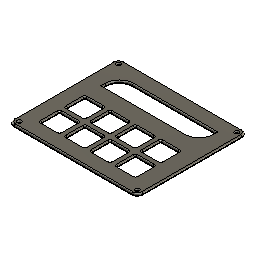
Final (Autodesk Fusion 360 archive; units mm, degrees)
design "Case_Lid"
Autodesk Fusion 360 part; units mm, degrees
(part 1 of 2)
sketch "plate-2025-12-06T19_36_10.325Z" plane through (0, 0, 0) normal (0, 0, 1) x (1, 0, 0)
  line L0 (3.275, -2.525) -> (15.775, -2.525)
  line L1 (3.275, -16.525) -> (15.775, -16.525)
  line L2 (2.525, -3.275) -> (2.525, -15.775)
  line L3 (16.525, -3.275) -> (16.525, -15.775)
  arc A0 (3.275, -2.525) -> (2.525, -3.275) centre (3.275, -3.275) ccw
  arc A1 (16.525, -3.275) -> (15.775, -2.525) centre (15.775, -3.275) ccw
  arc A2 (2.525, -15.775) -> (3.275, -16.525) centre (3.275, -15.775) ccw
  arc A3 (15.775, -16.525) -> (16.525, -15.775) centre (15.775, -15.775) ccw
  line L4 (22.325, -2.525) -> (34.825, -2.525)
  line L5 (22.325, -16.525) -> (34.825, -16.525)
  line L6 (21.575, -3.275) -> (21.575, -15.775)
  line L7 (35.575, -3.275) -> (35.575, -15.775)
  arc A4 (22.325, -2.525) -> (21.575, -3.275) centre (22.325, -3.275) ccw
  arc A5 (35.575, -3.275) -> (34.825, -2.525) centre (34.825, -3.275) ccw
  arc A6 (21.575, -15.775) -> (22.325, -16.525) centre (22.325, -15.775) ccw
  arc A7 (34.825, -16.525) -> (35.575, -15.775) centre (34.825, -15.775) ccw
  line L8 (41.375, -2.525) -> (53.875, -2.525)
  line L9 (41.375, -16.525) -> (53.875, -16.525)
  line L10 (40.625, -3.275) -> (40.625, -15.775)
  line L11 (54.625, -3.275) -> (54.625, -15.775)
  arc A8 (41.375, -2.525) -> (40.625, -3.275) centre (41.375, -3.275) ccw
  arc A9 (54.625, -3.275) -> (53.875, -2.525) centre (53.875, -3.275) ccw
  arc A10 (40.625, -15.775) -> (41.375, -16.525) centre (41.375, -15.775) ccw
  arc A11 (53.875, -16.525) -> (54.625, -15.775) centre (53.875, -15.775) ccw
  line L12 (60.425, -2.525) -> (72.925, -2.525)
  line L13 (60.425, -16.525) -> (72.925, -16.525)
  line L14 (59.675, -3.275) -> (59.675, -15.775)
  line L15 (73.675, -3.275) -> (73.675, -15.775)
  arc A12 (60.425, -2.525) -> (59.675, -3.275) centre (60.425, -3.275) ccw
  arc A13 (73.675, -3.275) -> (72.925, -2.525) centre (72.925, -3.275) ccw
  arc A14 (59.675, -15.775) -> (60.425, -16.525) centre (60.425, -15.775) ccw
  arc A15 (72.925, -16.525) -> (73.675, -15.775) centre (72.925, -15.775) ccw
  line L16 (3.275, -21.575) -> (15.775, -21.575)
  line L17 (3.275, -35.575) -> (15.775, -35.575)
  line L18 (2.525, -22.325) -> (2.525, -34.825)
  line L19 (16.525, -22.325) -> (16.525, -34.825)
  arc A16 (3.275, -21.575) -> (2.525, -22.325) centre (3.275, -22.325) ccw
  arc A17 (16.525, -22.325) -> (15.775, -21.575) centre (15.775, -22.325) ccw
  arc A18 (2.525, -34.825) -> (3.275, -35.575) centre (3.275, -34.825) ccw
  arc A19 (15.775, -35.575) -> (16.525, -34.825) centre (15.775, -34.825) ccw
  line L20 (22.325, -21.575) -> (34.825, -21.575)
  line L21 (22.325, -35.575) -> (34.825, -35.575)
  line L22 (21.575, -22.325) -> (21.575, -34.825)
  line L23 (35.575, -22.325) -> (35.575, -34.825)
  arc A20 (22.325, -21.575) -> (21.575, -22.325) centre (22.325, -22.325) ccw
  arc A21 (35.575, -22.325) -> (34.825, -21.575) centre (34.825, -22.325) ccw
  arc A22 (21.575, -34.825) -> (22.325, -35.575) centre (22.325, -34.825) ccw
  arc A23 (34.825, -35.575) -> (35.575, -34.825) centre (34.825, -34.825) ccw
  line L24 (41.375, -21.575) -> (53.875, -21.575)
  line L25 (41.375, -35.575) -> (53.875, -35.575)
  line L26 (40.625, -22.325) -> (40.625, -34.825)
  line L27 (54.625, -22.325) -> (54.625, -34.825)
  arc A24 (41.375, -21.575) -> (40.625, -22.325) centre (41.375, -22.325) ccw
  arc A25 (54.625, -22.325) -> (53.875, -21.575) centre (53.875, -22.325) ccw
  arc A26 (40.625, -34.825) -> (41.375, -35.575) centre (41.375, -34.825) ccw
  arc A27 (53.875, -35.575) -> (54.625, -34.825) centre (53.875, -34.825) ccw
  line L28 (60.425, -21.575) -> (72.925, -21.575)
  line L29 (60.425, -35.575) -> (72.925, -35.575)
  line L30 (59.675, -22.325) -> (59.675, -34.825)
  line L31 (73.675, -22.325) -> (73.675, -34.825)
  arc A28 (60.425, -21.575) -> (59.675, -22.325) centre (60.425, -22.325) ccw
  arc A29 (73.675, -22.325) -> (72.925, -21.575) centre (72.925, -22.325) ccw
  arc A30 (59.675, -34.825) -> (60.425, -35.575) centre (60.425, -34.825) ccw
  arc A31 (72.925, -35.575) -> (73.675, -34.825) centre (72.925, -34.825) ccw
  line L32 (-9.861, 35.425) -> (87.139, 35.425)
  line L33 (87.139, 35.425) -> (87.139, -47.575)
  line L34 (87.139, -47.575) -> (-9.861, -47.575)
  line L35 (-9.861, -47.575) -> (-9.861, 35.425)
  line L36 (12.525, 23.425) -> (74.753, 23.425)
  line L37 (74.753, 23.425) -> (74.753, 21.425)
  line L38 (64.753, 11.425) -> (2.525, 11.425)
  line L39 (2.525, 11.425) -> (2.525, 13.425)
  arc A32 (12.525, 23.425) -> (2.525, 13.425) centre (12.525, 13.425) ccw
  arc A33 (64.753, 11.425) -> (74.753, 21.425) centre (64.753, 21.425) ccw
  circle A34 centre (-5.861, 31.425) radius 1.6
  circle A35 centre (83.139, 31.425) radius 1.6
  circle A36 centre (83.139, -43.575) radius 1.6
  circle A37 centre (-5.861, -43.575) radius 1.6
  point P0 (74.753, 11.425)
  dimension "d1" = 97
  dimension "d2" = 83
  dimension "d3" = 12.386
  dimension "d4" = 12
  dimension "d5" = 0
  dimension "d6" = 12.386
  dimension "d7" = 12.386
  dimension "d8" = 12
  dimension "d9" = 12
  dimension "d10" = 10
  dimension "d11" = 10
  dimension "d12" = 3.2
  dimension "d13" = 4
  dimension "d14" = 4
  dimension "d15" = 3.2
  dimension "d16" = 4
  dimension "d17" = 4
  dimension "d18" = 3.2
  dimension "d19" = 3.2
  dimension "d20" = 4
  dimension "d21" = 4
  dimension "d22" = 4
  dimension "d23" = 4
  constraint horizontal L32
  constraint vertical L33
  constraint horizontal L34
  constraint vertical L35
  constraint horizontal L36
  constraint vertical L37
  constraint horizontal L38
  constraint vertical L39
  constraint tangent L36 A32
  constraint tangent L39 A32
  constraint coincident P0 L38
  constraint tangent L37 A33
  constraint tangent L38 A33
  measures "d1" distance of L32.start L32.end
  measures "d2" distance of L32.start L34.end
  measures "d3" distance of L18 L35
  measures "d4" distance of L17 L34
  measures "d5" distance of L2 L39
  measures "d6" distance of L33 L37
  measures "d7" distance of L35 L39
  measures "d8" distance of L36.end P0
  measures "d9" distance of L32 L36
  measures "d10" radius of A32
  measures "d11" radius of A33
  measures "d12" diameter of A34
  measures "d13" distance of L32 A34.centre
  measures "d14" distance of L35 A34.centre
  measures "d15" diameter of A35
  measures "d16" distance of L33 A35.centre
  measures "d17" distance of L32 A35.centre
  measures "d18" diameter of A37
  measures "d19" diameter of A36
  measures "d20" distance of L34 A36.centre
  measures "d21" distance of L33 A36.centre
  measures "d22" distance of L34 A37.centre
  measures "d23" distance of L35 A37.centre
extrude "Extrude1" add sketch "plate-2025-12-06T19_36_10.325Z" along normal blind 1.5
fillet "Fillet2" radius 4.3 4 edges at (-9.861, 35.425, 0.75) (87.139, 35.425, 0.75) (-9.861, -47.575, 0.75) (87.139, -47.575, 0.75)
fillet "Fillet1" radius 1 74 edges at (21.7947, -35.3553, 1.5) (21.575, -28.575, 1.5) (21.7947, -21.7947, 1.5) (28.575, -21.575, 1.5) (35.3553, -21.7947, 1.5) (35.575, -28.575, 1.5) (35.3553, -35.3553, 1.5) (28.575, -35.575, 1.5) (2.525, -28.575, 1.5) (2.7447, -21.7947, 1.5) (9.525, -21.575, 1.5) (16.3053, -21.7947, 1.5) (16.525, -28.575, 1.5) (16.3053, -35.3553, 1.5) (9.525, -35.575, 1.5) (2.7447, -35.3553, 1.5) (28.575, -2.525, 1.5) (35.3553, -2.7447, 1.5) (35.575, -9.525, 1.5) (35.3553, -16.3053, 1.5) (28.575, -16.525, 1.5) (21.7947, -16.3053, 1.5) (21.575, -9.525, 1.5) (21.7947, -2.7447, 1.5) (74.753, 22.425, 1.5) (71.8241, 14.3539, 1.5) (33.639, 11.425, 1.5) (2.525, 12.425, 1.5) (5.4539, 20.4961, 1.5) (43.639, 23.425, 1.5) (87.139, -6.075, 1.5) (38.639, 35.425, 1.5) (-9.861, -6.075, 1.5) (38.639, -47.575, 1.5) (16.3053, -2.7447, 1.5) (16.525, -9.525, 1.5) (16.3053, -16.3053, 1.5) (9.525, -16.525, 1.5) (2.7447, -16.3053, 1.5) (2.525, -9.525, 1.5) (2.7447, -2.7447, 1.5) (9.525, -2.525, 1.5) (40.8447, -35.3553, 1.5) (40.625, -28.575, 1.5) (40.8447, -21.7947, 1.5) (47.625, -21.575, 1.5) (54.4053, -21.7947, 1.5) (54.625, -28.575, 1.5) (54.4053, -35.3553, 1.5) (47.625, -35.575, 1.5) (47.625, -2.525, 1.5) (54.4053, -2.7447, 1.5) (54.625, -9.525, 1.5) (54.4053, -16.3053, 1.5) (47.625, -16.525, 1.5) (40.8447, -16.3053, 1.5) (40.625, -9.525, 1.5) (40.8447, -2.7447, 1.5) (59.675, -9.525, 1.5) (59.8947, -2.7447, 1.5) (66.675, -2.525, 1.5) (73.4553, -2.7447, 1.5) (73.675, -9.525, 1.5) (73.4553, -16.3053, 1.5) (66.675, -16.525, 1.5) (59.8947, -16.3053, 1.5) (59.8947, -35.3553, 1.5) (59.675, -28.575, 1.5) (59.8947, -21.7947, 1.5) (66.675, -21.575, 1.5) (73.4553, -21.7947, 1.5) (73.675, -28.575, 1.5) (73.4553, -35.3553, 1.5) (66.675, -35.575, 1.5)
equation "d1 = 8 mm + 8 mm + 81 mm"
equation "d2 = 8 mm + 8 mm + 67 mm"
equation "d3 = 8 mm + 4.386 mm"
equation "d4 = 8 mm + 4 mm"

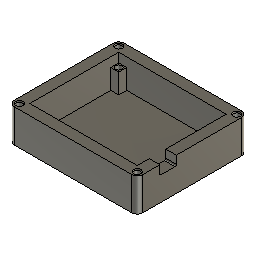
design "Case_Base"
Autodesk Fusion 360 part; units mm, degrees
sketch "Sketch1" plane through (0, 0, 0) normal (0, 0, 1) x (1, 0, 0) in component "Hackpad Case"
  line L0 (1, 47.0118) -> (82, 47.0118)
  line L1 (82, 47.0118) -> (82, -19.9882)
  line L2 (82, -19.9882) -> (1, -19.9882)
  line L3 (1, -19.9882) -> (1, 47.0118)
  line L4 (-7, 55.0118) -> (90, 55.0118)
  line L5 (90, 55.0118) -> (90, -27.9882)
  line L6 (90, -27.9882) -> (-7, -27.9882)
  line L7 (-7, -27.9882) -> (-7, 55.0118)
  circle A0 centre (-3, 51.0118) radius 2.35
  circle A1 centre (86, 51.0118) radius 2.35
  circle A2 centre (-3, -23.9882) radius 2.35
  circle A3 centre (86, -23.9882) radius 2.35
  circle A4 centre (4, 44.0118) radius 2.35
  line L8 (1, 47.0118) -> (7, 47.0118)
  line L9 (7, 47.0118) -> (7, 41.0118)
  line L10 (7, 41.0118) -> (1, 41.0118)
  line L11 (1, 41.0118) -> (1, 47.0118)
  circle A5 centre (79, 44.0118) radius 2.35
  line L12 (82, 47.0118) -> (76, 47.0118)
  line L13 (76, 47.0118) -> (76, 41.0118)
  line L14 (76, 41.0118) -> (82, 41.0118)
  line L15 (82, 41.0118) -> (82, 47.0118)
  circle A6 centre (4, -16.9882) radius 2.35
  line L16 (1, -19.9882) -> (7, -19.9882)
  line L17 (7, -19.9882) -> (7, -13.9882)
  line L18 (7, -13.9882) -> (1, -13.9882)
  line L19 (1, -13.9882) -> (1, -19.9882)
  line L20 (82, -19.9882) -> (76, -19.9882)
  line L21 (76, -19.9882) -> (76, -13.9882)
  line L22 (76, -13.9882) -> (82, -13.9882)
  line L23 (82, -13.9882) -> (82, -19.9882)
  circle A7 centre (79, -16.9882) radius 2.35
  point P0 (-24.0837, 40.5707)
  dimension "d1" = 81
  dimension "d2" = 67
  dimension "d3" = 8
  dimension "d4" = 8
  dimension "d5" = 8
  dimension "d6" = 8
  dimension "d7" = 4.7
  dimension "d8" = 4
  dimension "d9" = 4
  dimension "d10" = 4.7
  dimension "d11" = 4
  dimension "d12" = 4
  dimension "d13" = 4.7
  dimension "d14" = 4
  dimension "d15" = 4
  dimension "d16" = 4.7
  dimension "d17" = 4
  dimension "d18" = 4
  dimension "d22" = 4.7
  dimension "d23" = 3
  dimension "d24" = 3
  dimension "d25" = 6
  dimension "d26" = 6
  dimension "d27" = 4.7
  dimension "d28" = 6
  dimension "d29" = 6
  dimension "d30" = 3
  dimension "d31" = 3
  dimension "d32" = 4.7
  dimension "d33" = 6
  dimension "d34" = 6
  dimension "d35" = 3
  dimension "d36" = 3
  dimension "d37" = 6
  dimension "d38" = 6
  dimension "d39" = 4.7
  dimension "d40" = 3
  dimension "d41" = 3
  constraint horizontal L0
  constraint vertical L1
  constraint horizontal L2
  constraint vertical L3
  constraint horizontal L4
  constraint vertical L5
  constraint horizontal L6
  constraint vertical L7
  constraint horizontal L8
  constraint vertical L9
  constraint horizontal L10
  constraint vertical L11
  constraint horizontal L12
  constraint vertical L13
  constraint horizontal L14
  constraint vertical L15
  constraint horizontal L16
  constraint vertical L17
  constraint horizontal L18
  constraint vertical L19
  constraint horizontal L20
  constraint vertical L21
  constraint horizontal L22
  constraint vertical L23
  measures "d1" distance of L0.start L0.end
  measures "d2" distance of L0.start L2.end
  measures "d3" distance of L0 L4
  measures "d4" distance of L2 L6
  measures "d5" distance of L1 L5
  measures "d6" distance of L3 L7
  measures "d7" diameter of A0
  measures "d8" distance of L7 A0.centre
  measures "d9" distance of L4 A0.centre
  measures "d10" diameter of A1
  measures "d11" distance of L4 A1.centre
  measures "d12" distance of L5 A1.centre
  measures "d13" diameter of A2
  measures "d14" distance of L7 A2.centre
  measures "d15" distance of L6 A2.centre
  measures "d16" diameter of A3
  measures "d17" distance of L5 A3.centre
  measures "d18" distance of L6 A3.centre
  measures "d22" diameter of A4
  measures "d23" distance of L3 A4.centre
  measures "d24" distance of L0 A4.centre
  measures "d25" distance of L8.end L9.end
  measures "d26" distance of L9.end L10.end
  measures "d27" diameter of A5
  measures "d28" distance of L13.end L14.end
  measures "d29" distance of L12.end L13.end
  measures "d30" distance of A5.centre L12
  measures "d31" distance of L1 A5.centre
  measures "d32" diameter of A6
  measures "d33" distance of L17.end L18.end
  measures "d34" distance of L16.end L17.end
  measures "d35" distance of L2 A6.centre
  measures "d36" distance of A6.centre L19
  measures "d37" distance of L21.end L22.end
  measures "d38" distance of L20.end L21.end
  measures "d39" diameter of A7
  measures "d40" distance of L23 A7.centre
  measures "d41" distance of L2 A7.centre
extrude "Extrude1" add sketch "Sketch1" along normal blind 3.1 contours L0 L3 L8 L9 L10 L11 | L0 L1 L2 L3 L9 L10 L13 L14 L17 L18 L21 L22 | L0 L1 L12 L13 L14 L15 | L2 L3 L16 L17 L18 L19 | L1 L2 L20 L21 L22 L23 | L4 L5 L6 L7 | A0 | A1 | A2 | A3 | A4 | A5 | A6 | A7 in component "Hackpad Case"
extrude "Extrude2" add sketch "Sketch1" along normal blind 25 contours L4 L5 L6 L7 in component "Hackpad Case"
extrude "Extrude3" add sketch "Sketch1" along normal blind 18 contours L0 L3 L8 L9 L10 L11 | L0 L1 L12 L13 L14 L15 | L2 L3 L16 L17 L18 L19 | L1 L2 L20 L21 L22 L23 in component "Hackpad Case"
fillet "Fillet1" radius 4.3 4 edges at (90, -27.9882, 12.5) (90, 55.0118, 12.5) (-7, -27.9882, 12.5) (-7, 55.0118, 12.5) in component "Hackpad Case"
sketch "Sketch2" plane through (0, 0, 25) normal (0, 0, 1) x (-1, 0, 0) in component "Hackpad Case"
  circle A0 centre (3, 23.9882) radius 2.35
  circle A1 centre (3, -51.0118) radius 2.35
  line L0 (-82, -47.0118) -> (-82, 19.9882)
  line L1 (-82, 19.9882) -> (-1, 19.9882)
  line L2 (-1, 19.9882) -> (-1, -47.0118)
  line L3 (-1, -47.0118) -> (-82, -47.0118)
  circle A2 centre (-86, -51.0118) radius 2.35
  circle A3 centre (-86, 23.9882) radius 2.35
  arc A4 (2.7, -55.0118) -> (7, -50.7118) centre (2.7, -50.7118) ccw
  line L4 (7, -50.7118) -> (7, 23.6882)
  arc A5 (7, 23.6882) -> (2.7, 27.9882) centre (2.7, 23.6882) ccw
  line L5 (2.7, 27.9882) -> (-85.7, 27.9882)
  arc A6 (-85.7, 27.9882) -> (-90, 23.6882) centre (-85.7, 23.6882) ccw
  line L6 (-90, 23.6882) -> (-90, -50.7118)
  arc A7 (-90, -50.7118) -> (-85.7, -55.0118) centre (-85.7, -50.7118) ccw
  line L7 (-85.7, -55.0118) -> (2.7, -55.0118)
  line L8 (-82, -1.5118) -> (-90, -1.5118)
  line L9 (-90, -1.5118) -> (-90, 10.9882)
  line L10 (-90, 10.9882) -> (-82, 10.9882)
  line L11 (-82, 10.9882) -> (-82, -1.5118)
  dimension "d54" = 9
  dimension "d55" = 12.5
  constraint horizontal L8
  constraint vertical L9
  constraint horizontal L10
  constraint vertical L11
  constraint coincident L6 L9.end
  constraint coincident L0 L8.start
  measures "d54" distance of L1 L10
  measures "d55" distance of L8.end L9.end
extrude "Extrude4" cut sketch "Sketch2" against normal up to surface (7 mm away) contours L0 L6 L8 L9 L10 L11 in component "Hackpad Case"
fillet "Fillet2" radius 1 2 edges at (86, -10.9882, 18) (86, 1.5118, 18) in component "Hackpad Case"
chamfer "Chamfer1" distance 0.4 distance2 0.8 4 edges at (-5.191, -23.1384, 25) (-5.191, 51.8616, 25) (83.809, 51.8616, 25) (83.809, -23.1384, 25) measured on face at (84.6667, 16.6784, 25) measured on face at (84.6667, 16.6784, 25) measured on face at (84.6667, 16.6784, 25) measured on face at (84.6667, 16.6784, 25) in component "Hackpad Case"
sketch "Sketch1 (2)" plane through (0, 0, 0) normal (0, 0, -1) x (1, 0, 0)
  arc A0 (-7, -50.7118) -> (-2.7, -55.0118) centre (-2.7, -50.7118) ccw
  line L0 (-2.7, -55.0118) -> (85.7, -55.0118)
  arc A1 (85.7, -55.0118) -> (90, -50.7118) centre (85.7, -50.7118) ccw
  line L1 (90, -50.7118) -> (90, 23.6882)
  arc A2 (90, 23.6882) -> (85.7, 27.9882) centre (85.7, 23.6882) ccw
  line L2 (85.7, 27.9882) -> (-2.7, 27.9882)
  arc A3 (-2.7, 27.9882) -> (-7, 23.6882) centre (-2.7, 23.6882) ccw
  line L3 (-7, 23.6882) -> (-7, -50.7118)
  line L4 (86.6421, -50.8903) -> (39.0171, -50.8903)
  line L5 (39.0171, -50.8903) -> (39.0171, -35.0153)
  line L6 (39.0171, -35.0153) -> (86.6421, -35.0153)
  line L7 (86.6421, -35.0153) -> (86.6421, -50.8903)
  line L8 (54.9424, -39.6039) -> (57.298, -40.1975)
  line L9 (57.298, -40.1975) -> (57.2281, -40.4746)
  line L10 (57.2281, -40.4746) -> (54.7859, -39.859)
  spline S0 degree 3 poles (54.7859, -39.859) (54.5214, -40.2569) (54.1891, -40.6039) (53.7828, -40.8953) knots 0 0 0 0 1 1 1 1
  line L11 (53.7828, -40.8953) -> (53.1572, -43.2146)
  line L12 (53.1572, -43.2146) -> (51.4906, -41.7411)
  spline S1 degree 3 poles (51.4906, -41.7411) (49.6525, -42.1963) (47.9026, -42.1789) (46.2353, -41.7201) knots 0 0 0 0 1 1 1 1
  line L13 (46.2353, -41.7201) -> (44.5832, -43.0742)
  line L14 (44.5832, -43.0742) -> (44.2797, -41.1871)
  spline S2 degree 3 poles (44.2797, -41.1871) (43.932, -40.8137) (43.6708, -40.4314) (43.4786, -40.0419) knots 0 0 0 0 1 1 1 1
  line L15 (43.4786, -40.0419) -> (42.3068, -40.4518)
  line L16 (42.3068, -40.4518) -> (42.2124, -40.1822)
  line L17 (42.2124, -40.1822) -> (43.3603, -39.7805)
  spline S3 degree 3 poles (43.3603, -39.7805) (43.2125, -39.4227) (43.1191, -39.0592) (43.067, -38.6915) knots 0 0 0 0 1 1 1 1
  line L18 (43.067, -38.6915) -> (40.8577, -38.6743)
  line L19 (40.8577, -38.6743) -> (40.8598, -38.3886)
  line L20 (40.8598, -38.3886) -> (43.0346, -38.4054)
  spline S4 degree 3 poles (43.0346, -38.4054) (43.0153, -38.1788) (43.0102, -37.9506) (43.0164, -37.7212) knots 0 0 0 0 1 1 1 1
  line L21 (43.0164, -37.7212) -> (43.0203, -37.5772)
  line L22 (43.0203, -37.5772) -> (43.3083, -37.585)
  line L23 (43.3083, -37.585) -> (43.3044, -37.729)
  spline S5 degree 3 poles (43.3044, -37.729) (43.2982, -37.9566) (43.3038, -38.1829) (43.3244, -38.4077) knots 0 0 0 0 1 1 1 1
  line L24 (43.3244, -38.4077) -> (45.1702, -38.4221)
  line L25 (45.1702, -38.4221) -> (45.168, -38.7078)
  line L26 (45.168, -38.7078) -> (43.3591, -38.6938)
  spline S6 degree 3 poles (43.3591, -38.6938) (43.41, -39.0283) (43.498, -39.359) (43.6339, -39.6848) knots 0 0 0 0 1 1 1 1
  line L27 (43.6339, -39.6848) -> (45.2416, -39.1224)
  line L28 (45.2416, -39.1224) -> (45.336, -39.3921)
  line L29 (45.336, -39.3921) -> (43.7538, -39.9456)
  spline S7 degree 3 poles (43.7538, -39.9456) (43.9379, -40.3117) (44.1878, -40.671) (44.5195, -41.0217) knots 0 0 0 0 1 1 1 1
  line L30 (44.5195, -41.0217) -> (44.55, -41.0539)
  line L31 (44.55, -41.0539) -> (44.788, -42.5338)
  line L32 (44.788, -42.5338) -> (46.1689, -41.4022)
  line L33 (46.1689, -41.4022) -> (46.2413, -41.4227)
  spline S8 degree 3 poles (46.2413, -41.4227) (47.9053, -41.894) (49.6541, -41.911) (51.4936, -41.4433) knots 0 0 0 0 1 1 1 1
  line L34 (51.4936, -41.4433) -> (51.5675, -41.4245)
  line L35 (51.5675, -41.4245) -> (53, -42.6911)
  line L36 (53, -42.6911) -> (53.5317, -40.7195)
  line L37 (53.5317, -40.7195) -> (53.5747, -40.6895)
  spline S9 degree 3 poles (53.5747, -40.6895) (53.9407, -40.434) (54.2431, -40.1306) (54.4875, -39.7839) knots 0 0 0 0 1 1 1 1
  line L38 (54.4875, -39.7839) -> (53.0484, -39.4212)
  line L39 (53.0484, -39.4212) -> (53.1182, -39.144)
  line L40 (53.1182, -39.144) -> (54.6514, -39.5305)
  spline S10 degree 3 poles (54.6514, -39.5305) (54.8036, -39.2737) (54.9279, -38.9961) (55.0266, -38.6993) knots 0 0 0 0 1 1 1 1
  line L41 (55.0266, -38.6993) -> (53.8649, -38.9048)
  line L42 (53.8649, -38.9048) -> (53.8152, -38.6233)
  line L43 (53.8152, -38.6233) -> (55.1177, -38.393)
  spline S11 degree 3 poles (55.1177, -38.393) (55.1323, -38.3375) (55.1461, -38.2814) (55.1591, -38.2248) knots 0 0 0 0 1 1 1 1
  line L44 (55.1591, -38.2248) -> (55.1915, -38.0844)
  line L45 (55.1915, -38.0844) -> (55.4722, -38.1489)
  line L46 (55.4722, -38.1489) -> (55.44, -38.2894)
  spline S12 degree 3 poles (55.44, -38.2894) (55.4362, -38.3056) (55.4323, -38.3218) (55.4285, -38.338) knots 0 0 0 0 1 1 1 1
  line L47 (55.4285, -38.338) -> (56.726, -38.1084)
  line L48 (56.726, -38.1084) -> (56.7757, -38.3898)
  line L49 (56.7757, -38.3898) -> (55.3467, -38.6427)
  spline S13 degree 3 poles (55.3467, -38.6427) (55.2437, -38.9867) (55.1096, -39.3077) (54.9424, -39.6039) knots 0 0 0 0 1 1 1 1
  spline S14 degree 3 poles (82.8096, -44.1615) (83.112, -44.1615) (83.3711, -44.2087) (83.5869, -44.303) knots 0 0 0 0 1 1 1 1
  spline S15 degree 3 poles (83.5869, -44.303) (83.8028, -44.3974) (83.9627, -44.5346) (84.0667, -44.7146) knots 0 0 0 0 1 1 1 1
  spline S16 degree 3 poles (84.0667, -44.7146) (84.1707, -44.8947) (84.207, -45.1131) (84.1755, -45.3701) knots 0 0 0 0 1 1 1 1
  line L50 (84.1755, -45.3701) -> (83.486, -45.3701)
  spline S17 degree 3 poles (83.486, -45.3701) (83.5035, -45.1656) (83.4431, -45.0127) (83.3051, -44.9113) knots 0 0 0 0 1 1 1 1
  spline S18 degree 3 poles (83.3051, -44.9113) (83.167, -44.81) (82.9878, -44.7593) (82.7676, -44.7593) knots 0 0 0 0 1 1 1 1
  spline S19 degree 3 poles (82.7676, -44.7593) (82.5369, -44.7593) (82.3399, -44.8108) (82.1764, -44.9139) knots 0 0 0 0 1 1 1 1
  spline S20 degree 3 poles (82.1764, -44.9139) (82.013, -45.017) (81.9173, -45.1534) (81.8894, -45.3229) knots 0 0 0 0 1 1 1 1
  spline S21 degree 3 poles (81.8894, -45.3229) (81.8632, -45.475) (81.9082, -45.5895) (82.0244, -45.6664) knots 0 0 0 0 1 1 1 1
  spline S22 degree 3 poles (82.0244, -45.6664) (82.1406, -45.7432) (82.301, -45.8096) (82.5055, -45.8656) knots 0 0 0 0 1 1 1 1
  line L51 (82.5055, -45.8656) -> (82.9302, -45.9809)
  spline S23 degree 3 poles (82.9302, -45.9809) (83.229, -46.0596) (83.4594, -46.1823) (83.621, -46.3493) knots 0 0 0 0 1 1 1 1
  spline S24 degree 3 poles (83.621, -46.3493) (83.7827, -46.5162) (83.8408, -46.7422) (83.7954, -47.027) knots 0 0 0 0 1 1 1 1
  spline S25 degree 3 poles (83.7954, -47.027) (83.7586, -47.2577) (83.6682, -47.4596) (83.524, -47.6326) knots 0 0 0 0 1 1 1 1
  spline S26 degree 3 poles (83.524, -47.6326) (83.3798, -47.8057) (83.1958, -47.9403) (82.9722, -48.0364) knots 0 0 0 0 1 1 1 1
  spline S27 degree 3 poles (82.9722, -48.0364) (82.7484, -48.1325) (82.4993, -48.1806) (82.225, -48.1806) knots 0 0 0 0 1 1 1 1
  spline S28 degree 3 poles (82.225, -48.1806) (81.9505, -48.1806) (81.7124, -48.1325) (81.5105, -48.0364) knots 0 0 0 0 1 1 1 1
  spline S29 degree 3 poles (81.5105, -48.0364) (81.3086, -47.9403) (81.1579, -47.8079) (81.0582, -47.6391) knots 0 0 0 0 1 1 1 1
  spline S30 degree 3 poles (81.0582, -47.6391) (80.9587, -47.4706) (80.9245, -47.2769) (80.956, -47.0585) knots 0 0 0 0 1 1 1 1
  line L52 (80.956, -47.0585) -> (81.6324, -47.0585)
  spline S31 degree 3 poles (81.6324, -47.0585) (81.6219, -47.2245) (81.6753, -47.3538) (81.7923, -47.4465) knots 0 0 0 0 1 1 1 1
  spline S32 degree 3 poles (81.7923, -47.4465) (81.9095, -47.5392) (82.0738, -47.5855) (82.2852, -47.5855) knots 0 0 0 0 1 1 1 1
  spline S33 degree 3 poles (82.2852, -47.5855) (82.5072, -47.5855) (82.6885, -47.5369) (82.8292, -47.4399) knots 0 0 0 0 1 1 1 1
  spline S34 degree 3 poles (82.8292, -47.4399) (82.9699, -47.343) (83.0534, -47.221) (83.0796, -47.0742) knots 0 0 0 0 1 1 1 1
  spline S35 degree 3 poles (83.0796, -47.0742) (83.0989, -46.9658) (83.0809, -46.8767) (83.0258, -46.8068) knots 0 0 0 0 1 1 1 1
  spline S36 degree 3 poles (83.0258, -46.8068) (82.9708, -46.7369) (82.8957, -46.6805) (82.8004, -46.6377) knots 0 0 0 0 1 1 1 1
  spline S37 degree 3 poles (82.8004, -46.6377) (82.7052, -46.5948) (82.606, -46.5603) (82.5029, -46.5341) knots 0 0 0 0 1 1 1 1
  line L53 (82.5029, -46.5341) -> (82.1542, -46.4398)
  spline S38 degree 3 poles (82.1542, -46.4398) (81.9707, -46.3943) (81.7984, -46.3274) (81.6377, -46.2392) knots 0 0 0 0 1 1 1 1
  spline S39 degree 3 poles (81.6377, -46.2392) (81.4769, -46.1509) (81.3528, -46.0325) (81.2654, -45.8839) knots 0 0 0 0 1 1 1 1
  spline S40 degree 3 poles (81.2654, -45.8839) (81.1779, -45.7354) (81.1535, -45.5466) (81.192, -45.3177) knots 0 0 0 0 1 1 1 1
  spline S41 degree 3 poles (81.192, -45.3177) (81.2479, -44.9733) (81.4148, -44.6945) (81.6928, -44.4814) knots 0 0 0 0 1 1 1 1
  spline S42 degree 3 poles (81.6928, -44.4814) (81.9707, -44.2681) (82.3429, -44.1615) (82.8096, -44.1615) knots 0 0 0 0 1 1 1 1
  line L54 (79.383, -48.1282) -> (80.0305, -44.2218)
  line L55 (80.0305, -44.2218) -> (80.7306, -44.2218)
  line L56 (80.7306, -44.2218) -> (80.0829, -48.1282)
  line L57 (80.0829, -48.1282) -> (79.383, -48.1282)
  line L58 (79.244, -44.2218) -> (78.5965, -48.1282)
  line L59 (78.5965, -48.1282) -> (77.8964, -48.1282)
  line L60 (77.8964, -48.1282) -> (78.447, -44.8117)
  line L61 (78.447, -44.8117) -> (76.722, -44.8117)
  line L62 (76.722, -44.8117) -> (76.8189, -44.2218)
  line L63 (76.8189, -44.2218) -> (79.244, -44.2218)
  line L64 (76.4702, -44.2218) -> (74.4593, -48.1282)
  line L65 (74.4593, -48.1282) -> (73.5706, -48.1282)
  line L66 (73.5706, -48.1282) -> (72.8234, -44.2218)
  line L67 (72.8234, -44.2218) -> (73.5628, -44.2218)
  line L68 (73.5628, -44.2218) -> (73.7332, -45.1891)
  line L69 (73.7332, -45.1891) -> (75.1961, -45.1891)
  line L70 (75.1961, -45.1891) -> (75.6758, -44.2218)
  line L71 (75.6758, -44.2218) -> (76.4702, -44.2218)
  line L72 (74.9155, -45.7528) -> (73.8327, -45.7528)
  line L73 (73.8327, -45.7528) -> (73.9193, -46.251)
  spline S43 degree 3 poles (73.9193, -46.251) (73.9455, -46.4205) (73.9721, -46.6167) (73.9993, -46.8396) knots 0 0 0 0 1 1 1 1
  spline S44 degree 3 poles (73.9993, -46.8396) (74.0263, -47.0624) (74.0538, -47.3101) (74.0819, -47.5828) knots 0 0 0 0 1 1 1 1
  spline S45 degree 3 poles (74.0819, -47.5828) (74.1937, -47.3171) (74.2981, -47.0733) (74.3951, -46.8514) knots 0 0 0 0 1 1 1 1
  spline S46 degree 3 poles (74.3951, -46.8514) (74.4921, -46.6294) (74.5835, -46.4292) (74.6691, -46.251) knots 0 0 0 0 1 1 1 1
  line L74 (74.6691, -46.251) -> (74.9155, -45.7528)
  spline S47 degree 3 poles (70.9462, -44.1615) (71.2486, -44.1615) (71.5077, -44.2087) (71.7236, -44.303) knots 0 0 0 0 1 1 1 1
  spline S48 degree 3 poles (71.7236, -44.303) (71.9394, -44.3974) (72.0994, -44.5346) (72.2034, -44.7146) knots 0 0 0 0 1 1 1 1
  spline S49 degree 3 poles (72.2034, -44.7146) (72.3073, -44.8947) (72.3436, -45.1131) (72.3121, -45.3701) knots 0 0 0 0 1 1 1 1
  line L75 (72.3121, -45.3701) -> (71.6226, -45.3701)
  spline S50 degree 3 poles (71.6226, -45.3701) (71.6401, -45.1656) (71.5798, -45.0127) (71.4418, -44.9113) knots 0 0 0 0 1 1 1 1
  spline S51 degree 3 poles (71.4418, -44.9113) (71.3037, -44.81) (71.1246, -44.7593) (70.9043, -44.7593) knots 0 0 0 0 1 1 1 1
  spline S52 degree 3 poles (70.9043, -44.7593) (70.6735, -44.7593) (70.4765, -44.8108) (70.313, -44.9139) knots 0 0 0 0 1 1 1 1
  spline S53 degree 3 poles (70.313, -44.9139) (70.1497, -45.017) (70.0539, -45.1534) (70.026, -45.3229) knots 0 0 0 0 1 1 1 1
  spline S54 degree 3 poles (70.026, -45.3229) (69.9998, -45.475) (70.0448, -45.5895) (70.161, -45.6664) knots 0 0 0 0 1 1 1 1
  spline S55 degree 3 poles (70.161, -45.6664) (70.2773, -45.7432) (70.4376, -45.8096) (70.6421, -45.8656) knots 0 0 0 0 1 1 1 1
  line L76 (70.6421, -45.8656) -> (71.0668, -45.9809)
  spline S56 degree 3 poles (71.0668, -45.9809) (71.3658, -46.0596) (71.596, -46.1823) (71.7577, -46.3493) knots 0 0 0 0 1 1 1 1
  spline S57 degree 3 poles (71.7577, -46.3493) (71.9193, -46.5162) (71.9774, -46.7422) (71.932, -47.027) knots 0 0 0 0 1 1 1 1
  spline S58 degree 3 poles (71.932, -47.027) (71.8953, -47.2577) (71.8049, -47.4596) (71.6606, -47.6326) knots 0 0 0 0 1 1 1 1
  spline S59 degree 3 poles (71.6606, -47.6326) (71.5164, -47.8057) (71.3325, -47.9403) (71.1088, -48.0364) knots 0 0 0 0 1 1 1 1
  spline S60 degree 3 poles (71.1088, -48.0364) (70.8851, -48.1325) (70.636, -48.1806) (70.3616, -48.1806) knots 0 0 0 0 1 1 1 1
  spline S61 degree 3 poles (70.3616, -48.1806) (70.0872, -48.1806) (69.849, -48.1325) (69.6471, -48.0364) knots 0 0 0 0 1 1 1 1
  spline S62 degree 3 poles (69.6471, -48.0364) (69.4453, -47.9403) (69.2946, -47.8079) (69.1949, -47.6391) knots 0 0 0 0 1 1 1 1
  spline S63 degree 3 poles (69.1949, -47.6391) (69.0953, -47.4706) (69.0612, -47.2769) (69.0927, -47.0585) knots 0 0 0 0 1 1 1 1
  line L77 (69.0927, -47.0585) -> (69.769, -47.0585)
  spline S64 degree 3 poles (69.769, -47.0585) (69.7586, -47.2245) (69.8119, -47.3538) (69.929, -47.4465) knots 0 0 0 0 1 1 1 1
  spline S65 degree 3 poles (69.929, -47.4465) (70.0461, -47.5392) (70.2104, -47.5855) (70.4219, -47.5855) knots 0 0 0 0 1 1 1 1
  spline S66 degree 3 poles (70.4219, -47.5855) (70.6439, -47.5855) (70.8252, -47.5369) (70.966, -47.4399) knots 0 0 0 0 1 1 1 1
  spline S67 degree 3 poles (70.966, -47.4399) (71.1066, -47.343) (71.1901, -47.221) (71.2163, -47.0742) knots 0 0 0 0 1 1 1 1
  spline S68 degree 3 poles (71.2163, -47.0742) (71.2355, -46.9658) (71.2176, -46.8767) (71.1626, -46.8068) knots 0 0 0 0 1 1 1 1
  spline S69 degree 3 poles (71.1626, -46.8068) (71.1075, -46.7369) (71.0323, -46.6805) (70.9371, -46.6377) knots 0 0 0 0 1 1 1 1
  spline S70 degree 3 poles (70.9371, -46.6377) (70.8418, -46.5948) (70.7426, -46.5603) (70.6395, -46.5341) knots 0 0 0 0 1 1 1 1
  line L78 (70.6395, -46.5341) -> (70.2908, -46.4398)
  spline S71 degree 3 poles (70.2908, -46.4398) (70.1073, -46.3943) (69.9352, -46.3274) (69.7743, -46.2392) knots 0 0 0 0 1 1 1 1
  spline S72 degree 3 poles (69.7743, -46.2392) (69.6135, -46.1509) (69.4894, -46.0325) (69.4021, -45.8839) knots 0 0 0 0 1 1 1 1
  spline S73 degree 3 poles (69.4021, -45.8839) (69.3147, -45.7354) (69.2902, -45.5466) (69.3286, -45.3177) knots 0 0 0 0 1 1 1 1
  spline S74 degree 3 poles (69.3286, -45.3177) (69.3846, -44.9733) (69.5515, -44.6945) (69.8294, -44.4814) knots 0 0 0 0 1 1 1 1
  spline S75 degree 3 poles (69.8294, -44.4814) (70.1073, -44.2681) (70.4796, -44.1615) (70.9462, -44.1615) knots 0 0 0 0 1 1 1 1
  line L79 (68.2642, -46.5472) -> (68.0754, -48.1282)
  line L80 (68.0754, -48.1282) -> (67.4017, -48.1282)
  line L81 (67.4017, -48.1282) -> (67.732, -46.5472)
  line L82 (67.732, -46.5472) -> (68.2642, -46.5472)
  line L83 (84.2201, -37.7252) -> (83.5726, -41.6315)
  line L84 (83.5726, -41.6315) -> (82.8594, -41.6315)
  line L85 (82.8594, -41.6315) -> (83.0534, -40.4727)
  line L86 (83.0534, -40.4727) -> (83.1897, -39.7123)
  spline S76 degree 3 poles (83.1897, -39.7123) (83.0849, -39.8382) (82.9756, -39.961) (82.862, -40.0808) knots 0 0 0 0 1 1 1 1
  spline S77 degree 3 poles (82.862, -40.0808) (82.7484, -40.2005) (82.6225, -40.3277) (82.4845, -40.4622) knots 0 0 0 0 1 1 1 1
  line L87 (82.4845, -40.4622) -> (81.2654, -41.6315)
  line L88 (81.2654, -41.6315) -> (80.3556, -41.6315)
  line L89 (80.3556, -41.6315) -> (82.1358, -39.9404)
  line L90 (82.1358, -39.9404) -> (80.977, -37.7252)
  line L91 (80.977, -37.7252) -> (81.753, -37.7252)
  line L92 (81.753, -37.7252) -> (82.6628, -39.5106)
  line L93 (82.6628, -39.5106) -> (83.313, -38.9102)
  line L94 (83.313, -38.9102) -> (83.5069, -37.7252)
  line L95 (83.5069, -37.7252) -> (84.2201, -37.7252)
  line L96 (80.4448, -37.7252) -> (79.7972, -41.6315)
  line L97 (79.7972, -41.6315) -> (77.2593, -41.6315)
  line L98 (77.2593, -41.6315) -> (77.359, -41.0442)
  line L99 (77.359, -41.0442) -> (79.1968, -41.0442)
  line L100 (79.1968, -41.0442) -> (79.3699, -39.9877)
  line L101 (79.3699, -39.9877) -> (77.6684, -39.9877)
  line L102 (77.6684, -39.9877) -> (77.7653, -39.4082)
  line L103 (77.7653, -39.4082) -> (79.4695, -39.4082)
  line L104 (79.4695, -39.4082) -> (79.6478, -38.3123)
  line L105 (79.6478, -38.3123) -> (77.7995, -38.3123)
  line L106 (77.7995, -38.3123) -> (77.8964, -37.7252)
  line L107 (77.8964, -37.7252) -> (80.4448, -37.7252)
  line L108 (75.9957, -37.7252) -> (75.744, -39.2378)
  line L109 (75.744, -39.2378) -> (76.79, -41.6315)
  line L110 (76.79, -41.6315) -> (76.0114, -41.6315)
  line L111 (76.0114, -41.6315) -> (75.5186, -40.3993)
  spline S78 degree 3 poles (75.5186, -40.3993) (75.48, -40.3032) (75.4456, -40.2101) (75.415, -40.1201) knots 0 0 0 0 1 1 1 1
  spline S79 degree 3 poles (75.415, -40.1201) (75.3844, -40.0301) (75.3569, -39.9309) (75.3324, -39.8225) knots 0 0 0 0 1 1 1 1
  spline S80 degree 3 poles (75.3324, -39.8225) (75.2712, -39.9343) (75.2109, -40.0352) (75.1515, -40.1253) knots 0 0 0 0 1 1 1 1
  spline S81 degree 3 poles (75.1515, -40.1253) (75.092, -40.2153) (75.0283, -40.3066) (74.9601, -40.3993) knots 0 0 0 0 1 1 1 1
  line L112 (74.9601, -40.3993) -> (74.0739, -41.6315)
  line L113 (74.0739, -41.6315) -> (73.2219, -41.6315)
  line L114 (73.2219, -41.6315) -> (75.0466, -39.2378)
  line L115 (75.0466, -39.2378) -> (75.2957, -37.7252)
  line L116 (75.2957, -37.7252) -> (75.9957, -37.7252)
  line L117 (73.3451, -37.7252) -> (72.6976, -41.6315)
  line L118 (72.6976, -41.6315) -> (71.2372, -41.6315)
  spline S82 degree 3 poles (71.2372, -41.6315) (70.9384, -41.6315) (70.6963, -41.576) (70.5111, -41.465) knots 0 0 0 0 1 1 1 1
  spline S83 degree 3 poles (70.5111, -41.465) (70.3257, -41.3541) (70.1964, -41.2011) (70.123, -41.0062) knots 0 0 0 0 1 1 1 1
  spline S84 degree 3 poles (70.123, -41.0062) (70.0496, -40.8113) (70.0338, -40.5898) (70.0758, -40.3416) knots 0 0 0 0 1 1 1 1
  spline S85 degree 3 poles (70.0758, -40.3416) (70.116, -40.0916) (70.2051, -39.8692) (70.3432, -39.6743) knots 0 0 0 0 1 1 1 1
  spline S86 degree 3 poles (70.3432, -39.6743) (70.4813, -39.4795) (70.6627, -39.3261) (70.8872, -39.2143) knots 0 0 0 0 1 1 1 1
  spline S87 degree 3 poles (70.8872, -39.2143) (71.1119, -39.1024) (71.3744, -39.0464) (71.6751, -39.0464) knots 0 0 0 0 1 1 1 1
  line L119 (71.6751, -39.0464) -> (72.4275, -39.0464)
  line L120 (72.4275, -39.0464) -> (72.6451, -37.7252)
  line L121 (72.6451, -37.7252) -> (73.3451, -37.7252)
  line L122 (72.3305, -39.6232) -> (71.6751, -39.6232)
  spline S88 degree 3 poles (71.6751, -39.6232) (71.4042, -39.6232) (71.1975, -39.6914) (71.0551, -39.8278) knots 0 0 0 0 1 1 1 1
  spline S89 degree 3 poles (71.0551, -39.8278) (70.9126, -39.964) (70.8247, -40.1345) (70.7916, -40.3389) knots 0 0 0 0 1 1 1 1
  spline S90 degree 3 poles (70.7916, -40.3389) (70.7565, -40.5452) (70.789, -40.7144) (70.8885, -40.8463) knots 0 0 0 0 1 1 1 1
  spline S91 degree 3 poles (70.8885, -40.8463) (70.9882, -40.9782) (71.1726, -41.0442) (71.4418, -41.0442) knots 0 0 0 0 1 1 1 1
  line L123 (71.4418, -41.0442) -> (72.0972, -41.0442)
  line L124 (72.0972, -41.0442) -> (72.3305, -39.6232)
  line L125 (70.574, -37.7252) -> (68.5631, -41.6315)
  line L126 (68.5631, -41.6315) -> (67.6744, -41.6315)
  line L127 (67.6744, -41.6315) -> (66.9272, -37.7252)
  line L128 (66.9272, -37.7252) -> (67.6664, -37.7252)
  line L129 (67.6664, -37.7252) -> (67.8368, -38.6925)
  line L130 (67.8368, -38.6925) -> (69.2997, -38.6925)
  line L131 (69.2997, -38.6925) -> (69.7795, -37.7252)
  line L132 (69.7795, -37.7252) -> (70.574, -37.7252)
  line L133 (69.0193, -39.2562) -> (67.9365, -39.2562)
  line L134 (67.9365, -39.2562) -> (68.023, -39.7543)
  spline S92 degree 3 poles (68.023, -39.7543) (68.0492, -39.9239) (68.0759, -40.1201) (68.1029, -40.3429) knots 0 0 0 0 1 1 1 1
  spline S93 degree 3 poles (68.1029, -40.3429) (68.1301, -40.5657) (68.1576, -40.8135) (68.1855, -41.0861) knots 0 0 0 0 1 1 1 1
  spline S94 degree 3 poles (68.1855, -41.0861) (68.2974, -40.8205) (68.4019, -40.5767) (68.4989, -40.3547) knots 0 0 0 0 1 1 1 1
  spline S95 degree 3 poles (68.4989, -40.3547) (68.5958, -40.1328) (68.6872, -39.9326) (68.7728, -39.7543) knots 0 0 0 0 1 1 1 1
  line L135 (68.7728, -39.7543) -> (69.0193, -39.2562)
  line L136 (64.9844, -37.7252) -> (66.4054, -37.7252)
  line L137 (66.4054, -37.7252) -> (65.7578, -41.6315)
  line L138 (65.7578, -41.6315) -> (64.4653, -41.6315)
  spline S96 degree 3 poles (64.4653, -41.6315) (64.0773, -41.6315) (63.7522, -41.5533) (63.49, -41.3968) knots 0 0 0 0 1 1 1 1
  spline S97 degree 3 poles (63.49, -41.3968) (63.2278, -41.2404) (63.0417, -41.0162) (62.9316, -40.7243) knots 0 0 0 0 1 1 1 1
  spline S98 degree 3 poles (62.9316, -40.7243) (62.8215, -40.4325) (62.8005, -40.0838) (62.8687, -39.6783) knots 0 0 0 0 1 1 1 1
  spline S99 degree 3 poles (62.8687, -39.6783) (62.9701, -39.0665) (63.1999, -38.5881) (63.5582, -38.2429) knots 0 0 0 0 1 1 1 1
  spline S100 degree 3 poles (63.5582, -38.2429) (63.9165, -37.8977) (64.3919, -37.7252) (64.9844, -37.7252) knots 0 0 0 0 1 1 1 1
  line L139 (65.6058, -38.3307) -> (65.0212, -38.3307)
  spline S101 degree 3 poles (65.0212, -38.3307) (64.1944, -38.3307) (63.7076, -38.7816) (63.5608, -39.6836) knots 0 0 0 0 1 1 1 1
  spline S102 degree 3 poles (63.5608, -39.6836) (63.4123, -40.5784) (63.7408, -41.0259) (64.5466, -41.0259) knots 0 0 0 0 1 1 1 1
  line L140 (64.5466, -41.0259) -> (65.1601, -41.0259)
  line L141 (65.1601, -41.0259) -> (65.6058, -38.3307)
  line L142 (57.4731, -48.1436) -> (57.4731, -45.3714)
  line L143 (57.4731, -45.3714) -> (57.7969, -45.3714)
  line L144 (57.7969, -45.3714) -> (57.7969, -47.7977)
  line L145 (57.7969, -47.7977) -> (57.7987, -47.7977)
  line L146 (57.7987, -47.7977) -> (58.489, -47.3399)
  line L147 (58.489, -47.3399) -> (58.489, -47.6822)
  line L148 (58.489, -47.6822) -> (57.7969, -48.1436)
  line L149 (57.7969, -48.1436) -> (57.4731, -48.1436)
  line L150 (57.0396, -45.3714) -> (57.0396, -45.6523)
  line L151 (57.0396, -45.6523) -> (56.0534, -46.5528)
  spline S103 degree 3 poles (56.0534, -46.5528) (55.9356, -46.6608) (55.8398, -46.7557) (55.766, -46.8375) knots 0 0 0 0 1 1 1 1
  spline S104 degree 3 poles (55.766, -46.8375) (55.6922, -46.9194) (55.638, -46.9995) (55.6032, -47.0775) knots 0 0 0 0 1 1 1 1
  spline S105 degree 3 poles (55.6032, -47.0775) (55.5685, -47.1557) (55.5511, -47.2419) (55.5511, -47.3362) knots 0 0 0 0 1 1 1 1
  spline S106 degree 3 poles (55.5511, -47.3362) (55.5511, -47.5074) (55.6017, -47.6426) (55.7027, -47.7418) knots 0 0 0 0 1 1 1 1
  spline S107 degree 3 poles (55.7027, -47.7418) (55.8038, -47.841) (55.9424, -47.8906) (56.1185, -47.8906) knots 0 0 0 0 1 1 1 1
  spline S108 degree 3 poles (56.1185, -47.8906) (56.3084, -47.8906) (56.4554, -47.8327) (56.5596, -47.7167) knots 0 0 0 0 1 1 1 1
  spline S109 degree 3 poles (56.5596, -47.7167) (56.6637, -47.6007) (56.7158, -47.4441) (56.7158, -47.2469) knots 0 0 0 0 1 1 1 1
  line L152 (56.7158, -47.2469) -> (57.0284, -47.2469)
  spline S110 degree 3 poles (57.0284, -47.2469) (57.0284, -47.4317) (56.9909, -47.5948) (56.9159, -47.7362) knots 0 0 0 0 1 1 1 1
  spline S111 degree 3 poles (56.9159, -47.7362) (56.8408, -47.8777) (56.735, -47.9883) (56.5986, -48.0683) knots 0 0 0 0 1 1 1 1
  spline S112 degree 3 poles (56.5986, -48.0683) (56.4622, -48.1484) (56.3028, -48.1883) (56.1205, -48.1883) knots 0 0 0 0 1 1 1 1
  spline S113 degree 3 poles (56.1205, -48.1883) (55.9468, -48.1883) (55.7936, -48.1527) (55.6608, -48.0814) knots 0 0 0 0 1 1 1 1
  spline S114 degree 3 poles (55.6608, -48.0814) (55.5281, -48.0101) (55.424, -47.9114) (55.3482, -47.7855) knots 0 0 0 0 1 1 1 1
  spline S115 degree 3 poles (55.3482, -47.7855) (55.2726, -47.6596) (55.2347, -47.5142) (55.2347, -47.3492) knots 0 0 0 0 1 1 1 1
  spline S116 degree 3 poles (55.2347, -47.3492) (55.2347, -47.1706) (55.2841, -47.0062) (55.3827, -46.8561) knots 0 0 0 0 1 1 1 1
  spline S117 degree 3 poles (55.3827, -46.8561) (55.4813, -46.7061) (55.6324, -46.5385) (55.8358, -46.3537) knots 0 0 0 0 1 1 1 1
  line L153 (55.8358, -46.3537) -> (56.5856, -45.6728)
  line L154 (56.5856, -45.6728) -> (56.5856, -45.669)
  line L155 (56.5856, -45.669) -> (55.2181, -45.669)
  line L156 (55.2181, -45.669) -> (55.2181, -45.3714)
  line L157 (55.2181, -45.3714) -> (57.0396, -45.3714)
  spline S118 degree 3 poles (54.6412, -45.3398) (54.7058, -45.3398) (54.7606, -45.3623) (54.8059, -45.4077) knots 0 0 0 0 1 1 1 1
  spline S119 degree 3 poles (54.8059, -45.4077) (54.8512, -45.453) (54.8738, -45.5079) (54.8738, -45.5723) knots 0 0 0 0 1 1 1 1
  spline S120 degree 3 poles (54.8738, -45.5723) (54.8738, -45.6381) (54.8512, -45.6933) (54.8059, -45.7379) knots 0 0 0 0 1 1 1 1
  spline S121 degree 3 poles (54.8059, -45.7379) (54.7606, -45.7826) (54.7058, -45.8049) (54.6412, -45.8049) knots 0 0 0 0 1 1 1 1
  spline S122 degree 3 poles (54.6412, -45.8049) (54.5755, -45.8049) (54.5203, -45.7826) (54.4756, -45.7379) knots 0 0 0 0 1 1 1 1
  spline S123 degree 3 poles (54.4756, -45.7379) (54.4311, -45.6933) (54.4087, -45.6381) (54.4087, -45.5723) knots 0 0 0 0 1 1 1 1
  spline S124 degree 3 poles (54.4087, -45.5723) (54.4087, -45.5079) (54.4311, -45.453) (54.4756, -45.4077) knots 0 0 0 0 1 1 1 1
  spline S125 degree 3 poles (54.4756, -45.4077) (54.5203, -45.3623) (54.5755, -45.3398) (54.6412, -45.3398) knots 0 0 0 0 1 1 1 1
  spline S126 degree 3 poles (53.1732, -45.3342) (53.3506, -45.3342) (53.51, -45.371) (53.6514, -45.4448) knots 0 0 0 0 1 1 1 1
  spline S127 degree 3 poles (53.6514, -45.4448) (53.7929, -45.5187) (53.9057, -45.6189) (53.99, -45.7454) knots 0 0 0 0 1 1 1 1
  spline S128 degree 3 poles (53.99, -45.7454) (54.0744, -45.8719) (54.1203, -46.0151) (54.1277, -46.1752) knots 0 0 0 0 1 1 1 1
  line L158 (54.1277, -46.1752) -> (53.7929, -46.1752)
  spline S129 degree 3 poles (53.7929, -46.1752) (53.7779, -46.0176) (53.7132, -45.8877) (53.5984, -45.7853) knots 0 0 0 0 1 1 1 1
  spline S130 degree 3 poles (53.5984, -45.7853) (53.4837, -45.683) (53.3419, -45.6319) (53.1732, -45.6319) knots 0 0 0 0 1 1 1 1
  spline S131 degree 3 poles (53.1732, -45.6319) (53.053, -45.6319) (52.9478, -45.6598) (52.8579, -45.7155) knots 0 0 0 0 1 1 1 1
  spline S132 degree 3 poles (52.8579, -45.7155) (52.768, -45.7714) (52.6975, -45.8481) (52.6467, -45.9453) knots 0 0 0 0 1 1 1 1
  spline S133 degree 3 poles (52.6467, -45.9453) (52.5958, -46.0427) (52.5704, -46.1541) (52.5704, -46.2793) knots 0 0 0 0 1 1 1 1
  spline S134 degree 3 poles (52.5704, -46.2793) (52.5704, -46.4046) (52.5947, -46.5157) (52.643, -46.6124) knots 0 0 0 0 1 1 1 1
  spline S135 degree 3 poles (52.643, -46.6124) (52.6914, -46.7092) (52.759, -46.7851) (52.8458, -46.8403) knots 0 0 0 0 1 1 1 1
  spline S136 degree 3 poles (52.8458, -46.8403) (52.9326, -46.8955) (53.0338, -46.9231) (53.1491, -46.9231) knots 0 0 0 0 1 1 1 1
  spline S137 degree 3 poles (53.1491, -46.9231) (53.3017, -46.9231) (53.4325, -46.8924) (53.5417, -46.8311) knots 0 0 0 0 1 1 1 1
  spline S138 degree 3 poles (53.5417, -46.8311) (53.6508, -46.7696) (53.727, -46.68) (53.7705, -46.5622) knots 0 0 0 0 1 1 1 1
  line L159 (53.7705, -46.5622) -> (54.0924, -46.5622)
  line L160 (54.0924, -46.5622) -> (53.9994, -48.1436)
  line L161 (53.9994, -48.1436) -> (52.3992, -48.1436)
  line L162 (52.3992, -48.1436) -> (52.3992, -47.846)
  line L163 (52.3992, -47.846) -> (53.6961, -47.846)
  line L164 (53.6961, -47.846) -> (53.763, -46.9473)
  line L165 (53.763, -46.9473) -> (53.7594, -46.9473)
  spline S139 degree 3 poles (53.7594, -46.9473) (53.5869, -47.1322) (53.3699, -47.2245) (53.1082, -47.2245) knots 0 0 0 0 1 1 1 1
  spline S140 degree 3 poles (53.1082, -47.2245) (52.9382, -47.2245) (52.7884, -47.1843) (52.6588, -47.1036) knots 0 0 0 0 1 1 1 1
  spline S141 degree 3 poles (52.6588, -47.1036) (52.5291, -47.023) (52.4281, -46.9119) (52.3555, -46.7705) knots 0 0 0 0 1 1 1 1
  spline S142 degree 3 poles (52.3555, -46.7705) (52.2829, -46.6292) (52.2467, -46.4666) (52.2467, -46.2831) knots 0 0 0 0 1 1 1 1
  spline S143 degree 3 poles (52.2467, -46.2831) (52.2467, -46.097) (52.2855, -45.9327) (52.3629, -45.7901) knots 0 0 0 0 1 1 1 1
  spline S144 degree 3 poles (52.3629, -45.7901) (52.4404, -45.6474) (52.5487, -45.5358) (52.6876, -45.4551) knots 0 0 0 0 1 1 1 1
  spline S145 degree 3 poles (52.6876, -45.4551) (52.8266, -45.3745) (52.9884, -45.3342) (53.1732, -45.3342) knots 0 0 0 0 1 1 1 1
  spline S146 degree 3 poles (51.7629, -45.3398) (51.8274, -45.3398) (51.8824, -45.3623) (51.9276, -45.4077) knots 0 0 0 0 1 1 1 1
  spline S147 degree 3 poles (51.9276, -45.4077) (51.9729, -45.453) (51.9955, -45.5079) (51.9955, -45.5723) knots 0 0 0 0 1 1 1 1
  spline S148 degree 3 poles (51.9955, -45.5723) (51.9955, -45.6381) (51.9729, -45.6933) (51.9276, -45.7379) knots 0 0 0 0 1 1 1 1
  spline S149 degree 3 poles (51.9276, -45.7379) (51.8824, -45.7826) (51.8274, -45.8049) (51.7629, -45.8049) knots 0 0 0 0 1 1 1 1
  spline S150 degree 3 poles (51.7629, -45.8049) (51.6972, -45.8049) (51.642, -45.7826) (51.5974, -45.7379) knots 0 0 0 0 1 1 1 1
  spline S151 degree 3 poles (51.5974, -45.7379) (51.5527, -45.6933) (51.5303, -45.6381) (51.5303, -45.5723) knots 0 0 0 0 1 1 1 1
  spline S152 degree 3 poles (51.5303, -45.5723) (51.5303, -45.5079) (51.5527, -45.453) (51.5974, -45.4077) knots 0 0 0 0 1 1 1 1
  spline S153 degree 3 poles (51.5974, -45.4077) (51.642, -45.3623) (51.6972, -45.3398) (51.7629, -45.3398) knots 0 0 0 0 1 1 1 1
  line L166 (51.1675, -45.3714) -> (51.1675, -45.6523)
  line L167 (51.1675, -45.6523) -> (50.1814, -46.5528)
  spline S154 degree 3 poles (50.1814, -46.5528) (50.0636, -46.6608) (49.9678, -46.7557) (49.894, -46.8375) knots 0 0 0 0 1 1 1 1
  spline S155 degree 3 poles (49.894, -46.8375) (49.8201, -46.9194) (49.7659, -46.9995) (49.7311, -47.0775) knots 0 0 0 0 1 1 1 1
  spline S156 degree 3 poles (49.7311, -47.0775) (49.6964, -47.1557) (49.679, -47.2419) (49.679, -47.3362) knots 0 0 0 0 1 1 1 1
  spline S157 degree 3 poles (49.679, -47.3362) (49.679, -47.5074) (49.7296, -47.6426) (49.8306, -47.7418) knots 0 0 0 0 1 1 1 1
  spline S158 degree 3 poles (49.8306, -47.7418) (49.9318, -47.841) (50.0704, -47.8906) (50.2465, -47.8906) knots 0 0 0 0 1 1 1 1
  spline S159 degree 3 poles (50.2465, -47.8906) (50.4363, -47.8906) (50.5833, -47.8327) (50.6875, -47.7167) knots 0 0 0 0 1 1 1 1
  spline S160 degree 3 poles (50.6875, -47.7167) (50.7916, -47.6007) (50.8438, -47.4441) (50.8438, -47.2469) knots 0 0 0 0 1 1 1 1
  line L168 (50.8438, -47.2469) -> (51.1563, -47.2469)
  spline S161 degree 3 poles (51.1563, -47.2469) (51.1563, -47.4317) (51.1188, -47.5948) (51.0438, -47.7362) knots 0 0 0 0 1 1 1 1
  spline S162 degree 3 poles (51.0438, -47.7362) (50.9687, -47.8777) (50.863, -47.9883) (50.7266, -48.0683) knots 0 0 0 0 1 1 1 1
  spline S163 degree 3 poles (50.7266, -48.0683) (50.5901, -48.1484) (50.4307, -48.1883) (50.2484, -48.1883) knots 0 0 0 0 1 1 1 1
  spline S164 degree 3 poles (50.2484, -48.1883) (50.0747, -48.1883) (49.9216, -48.1527) (49.7889, -48.0814) knots 0 0 0 0 1 1 1 1
  spline S165 degree 3 poles (49.7889, -48.0814) (49.6561, -48.0101) (49.5519, -47.9114) (49.4763, -47.7855) knots 0 0 0 0 1 1 1 1
  spline S166 degree 3 poles (49.4763, -47.7855) (49.4006, -47.6596) (49.3628, -47.5142) (49.3628, -47.3492) knots 0 0 0 0 1 1 1 1
  spline S167 degree 3 poles (49.3628, -47.3492) (49.3628, -47.1706) (49.412, -47.0062) (49.5106, -46.8561) knots 0 0 0 0 1 1 1 1
  spline S168 degree 3 poles (49.5106, -46.8561) (49.6093, -46.7061) (49.7603, -46.5385) (49.9637, -46.3537) knots 0 0 0 0 1 1 1 1
  line L169 (49.9637, -46.3537) -> (50.7136, -45.6728)
  line L170 (50.7136, -45.6728) -> (50.7136, -45.669)
  line L171 (50.7136, -45.669) -> (49.346, -45.669)
  line L172 (49.346, -45.669) -> (49.346, -45.3714)
  line L173 (49.346, -45.3714) -> (51.1675, -45.3714)
  spline S169 degree 3 poles (48.0194, -45.3267) (48.224, -45.3267) (48.4011, -45.3853) (48.5506, -45.5026) knots 0 0 0 0 1 1 1 1
  spline S170 degree 3 poles (48.5506, -45.5026) (48.7001, -45.6198) (48.8157, -45.785) (48.8976, -45.9984) knots 0 0 0 0 1 1 1 1
  spline S171 degree 3 poles (48.8976, -45.9984) (48.9795, -46.2118) (49.0204, -46.4641) (49.0204, -46.7557) knots 0 0 0 0 1 1 1 1
  spline S172 degree 3 poles (49.0204, -46.7557) (49.0204, -47.0484) (48.9795, -47.3017) (48.8976, -47.5158) knots 0 0 0 0 1 1 1 1
  spline S173 degree 3 poles (48.8976, -47.5158) (48.8157, -47.7297) (48.7001, -47.8953) (48.5506, -48.0125) knots 0 0 0 0 1 1 1 1
  spline S174 degree 3 poles (48.5506, -48.0125) (48.4011, -48.1297) (48.224, -48.1883) (48.0194, -48.1883) knots 0 0 0 0 1 1 1 1
  spline S175 degree 3 poles (48.0194, -48.1883) (47.8147, -48.1883) (47.6374, -48.1297) (47.4873, -48.0125) knots 0 0 0 0 1 1 1 1
  spline S176 degree 3 poles (47.4873, -48.0125) (47.3371, -47.8953) (47.2215, -47.7297) (47.1403, -47.5158) knots 0 0 0 0 1 1 1 1
  spline S177 degree 3 poles (47.1403, -47.5158) (47.059, -47.3017) (47.0184, -47.0484) (47.0184, -46.7557) knots 0 0 0 0 1 1 1 1
  spline S178 degree 3 poles (47.0184, -46.7557) (47.0184, -46.4641) (47.059, -46.2118) (47.1403, -45.9984) knots 0 0 0 0 1 1 1 1
  spline S179 degree 3 poles (47.1403, -45.9984) (47.2215, -45.785) (47.3371, -45.6198) (47.4873, -45.5026) knots 0 0 0 0 1 1 1 1
  spline S180 degree 3 poles (47.4873, -45.5026) (47.6374, -45.3853) (47.8147, -45.3267) (48.0194, -45.3267) knots 0 0 0 0 1 1 1 1
  spline S181 degree 3 poles (48.0194, -45.6244) (47.8073, -45.6244) (47.6402, -45.7252) (47.518, -45.9268) knots 0 0 0 0 1 1 1 1
  spline S182 degree 3 poles (47.518, -45.9268) (47.3958, -46.1283) (47.3347, -46.4046) (47.3347, -46.7557) knots 0 0 0 0 1 1 1 1
  spline S183 degree 3 poles (47.3347, -46.7557) (47.3347, -47.1092) (47.3958, -47.3867) (47.518, -47.5882) knots 0 0 0 0 1 1 1 1
  spline S184 degree 3 poles (47.518, -47.5882) (47.6402, -47.7898) (47.8073, -47.8906) (48.0194, -47.8906) knots 0 0 0 0 1 1 1 1